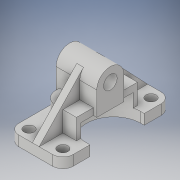
# Autodesk Inventor part: 模型2
Saved by Autodesk Inventor 2018 (Build 220112000, 112)
## iProperties
Created: 2020-05-06
Part Number: 模型2
Material: 常规
Document SubType Name: Modeling
Designer: PC
Density: 1 g/cm^3
Appearance: 默认
Author: PC
Autodesk Inventor part; units mm, degrees
ref_plane "YZ Plane" through (0, 0, 0) normal (1, 0, 0) x (0, 1, 0)
ref_plane "XZ Plane" through (0, 0, 0) normal (0, 1, 0) x (-1, 0, 0)
ref_plane "XY Plane" through (0, 0, 0) normal (0, 0, 1) x (1, 0, 0)
sketch "草图1" plane through (0, 0, 0) normal (0, 1, 0) x (-1, 0, 0)
  line L0 (-40, 80) -> (40, 80)
  line L1 (40, 80) -> (40, -80)
  line L2 (40, -80) -> (-40, -80)
  line L3 (-40, -80) -> (-40, 80)
  line L4 (-40, 80) -> (40, -80) construction
  line L5 (40, 80) -> (-40, -80) construction
  point P0 (0, 0)
  dimension "d0" = 160
  dimension "d1" = 80
  constraints: 12 end point, 2 midpoint, 2 parallel, 1 horizontal, 1 perpendicular
  measures "d0" distance of L0.end L1.end
  measures "d1" distance of L1.end L2.end
extrude "拉伸1" add sketch "草图1" along normal blind 15
sketch "草图2" plane through (0, 15, 0) normal (0, 1, 0) x (1, 0, 0)
  line L0 (25, -45) -> (-25, -45)
  line L1 (-25, -45) -> (-25, 45)
  line L2 (-25, 45) -> (25, 45)
  line L3 (25, 45) -> (25, -45)
  line L4 (25, -45) -> (-25, 45) construction
  line L5 (-25, -45) -> (25, 45) construction
  point P0 (0, 0)
  dimension "d4" = 90
  dimension "d5" = 50
  constraints: 12 end point, 2 midpoint, 2 parallel, 1 horizontal, 1 perpendicular
  measures "d4" distance of L0.end L1.end
  measures "d5" distance of L1.end L2.end
extrude "拉伸2" add sketch "草图2" along normal blind 30
sketch "草图3" plane through (0, 0, 0) normal (1, 0, 0) x (0, 1, 0)
  line L0 (0, 0) -> (70, 0) construction
  arc A0 (70, -20) -> (70, 20) centre (70, 0) ccw
  line L1 (70, 20) -> (15, 20)
  line L2 (15, -80) -> (15, 80) construction
  line L3 (70, -20) -> (15, -20)
  line L4 (15, -20) -> (15, 20)
  circle A1 centre (70, 0) radius 10
  line L5 (0, 80) -> (0, -80) projected
  dimension "d8" = 20
  dimension "d9" = 20
  dimension "d10" = 70
  constraints: 8 end point, 2 centre point, 2 coincident, 2 horizontal, 2 point on circle, 2 point on line, 2 tangent, 1 collinear, 1 perpendicular
  measures "d8" radius of A0
  measures "d9" diameter of A1
  measures "d10" distance from line of L5 A1.centre
extrude "拉伸3" add sketch "草图3" along normal mid plane 60
sketch "草图4" plane through (0, 15, 0) normal (0, 1, 0) x (1, 0, 0)
  line L0 (25, -65) -> (-25, -65) construction
  line L1 (-25, -65) -> (-25, 65) construction
  line L2 (-25, 65) -> (25, 65) construction
  line L3 (25, 65) -> (25, -65) construction
  line L4 (25, -65) -> (-25, 65) construction
  line L5 (-25, -65) -> (25, 65) construction
  circle A0 centre (-25, -65) radius 7.5
  circle A1 centre (-25, 65) radius 7.5
  circle A2 centre (25, 65) radius 7.5
  circle A3 centre (25, -65) radius 7.5
  point P0 (0, 0)
  dimension "d13" = 130
  dimension "d14" = 50
  dimension "d15" = 15
  constraints: 12 end point, 4 centre point, 4 coincident, 3 equal radius, 2 midpoint, 2 parallel, 1 horizontal, 1 perpendicular
  measures "d13" distance of L0.end L1.end
  measures "d14" distance of L1.end L2.end
  measures "d15" diameter of A0
extrude "拉伸4" cut sketch "草图4" against normal blind 60
fillet "圆角1" radius 15 4 edges at (40, 7.5, 80) (40, 7.5, -80) (-40, 7.5, 80) (-40, 7.5, -80)
fillet "圆角2" radius 20 2 edges at (-25, 30, -45) (-25, 30, 45)
sketch "草图5" plane through (0, 0, 0) normal (0, 1, 0) x (-1, 0, 0)
  line L0 (0, 0) -> (-35, 0) construction
  arc A0 (-35, -40) -> (-35, 40) centre (-35, 0) ccw
  line L1 (-40, 65) -> (-40, -65) construction
  line L2 (-35, 40) -> (-40, 40)
  line L3 (-40, 40) -> (-40, -40)
  line L4 (-40, -40) -> (-35, -40)
  dimension "d20" = 5
  dimension "d21" = 40
  constraints: 8 end point, 2 horizontal, 2 point on circle, 2 point on line, 2 tangent, 1 centre point, 1 coincident, 1 perpendicular
  measures "d20" distance from line of L1 L0.end
  measures "d21" radius of A0
extrude "拉伸5" cut sketch "草图5" along normal blind 35
sketch "草图6" plane through (0, 0, 0) normal (1, 0, 0) x (0, 1, 0)
  arc A0 (70, -20) -> (70, 20) centre (70, 0) ccw projected
  line L0 (70, 20) -> (35, 20) projected
  line L1 (45, 45) -> (45, 20) projected
  line L2 (15, 45) -> (45, 45) projected
  line L3 (15, 65) -> (15, 40) projected
  line L4 (15, 80) -> (15, 65) projected
  line L5 (15, 80) -> (83.7931, 14.4828)
  arc A1 (70, -20) -> (70, 20) centre (70, 0) ccw projected
  arc A2 (83.7931, 14.4828) -> (70, 20) centre (70, 0) ccw
  line L6 (45, 20) -> (45, 25) projected
  line L7 (70, 20) -> (45, 20)
  line L8 (45, 45) -> (45, 25) projected
  line L9 (45, 20) -> (45, 45)
  line L10 (15, 45) -> (45, 45) projected
  line L11 (45, 45) -> (15, 45)
  line L12 (15, 80) -> (15, 65) projected
  line L13 (15, 45) -> (15, 80)
  point P0 (0, 0)
  constraints: 10 end point, 3 point on circle, 1 centre point, 1 coincident, 1 collinear, 1 horizontal, 1 perpendicular, 1 tangent, 1 vertical
extrude "拉伸6" add sketch "草图6" along normal mid plane 10
mirror "镜像1" about plane through (0, 0, 0) normal (0, 0, 1) of "拉伸6"
